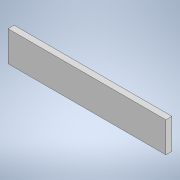
# Autodesk Inventor part: GroundShorttrack
Saved by Autodesk Inventor 2021 (Build 250183000, 183)
## iProperties
Created: 2022-07-02
Part Number: GroundShorttrack
Material: 一般
Document SubType Name: Modeling
Designer: tazak
Density: 1 g/cm^3
Appearance: 既定
Author: tazak
Autodesk Inventor part; units mm, degrees
ref_plane "YZ Plane" through (0, 0, 0) normal (1, 0, 0) x (0, 1, 0)
ref_plane "XZ Plane" through (0, 0, 0) normal (0, 1, 0) x (-1, 0, 0)
ref_plane "XY Plane" through (0, 0, 0) normal (0, 0, 1) x (1, 0, 0)
sketch "スケッチ1" plane through (0, 0, 0) normal (0, 0, 1) x (1, 0, 0)
  line L0 (-1000, 2500) -> (25000, 2500)
  line L1 (25000, 2500) -> (25000, -2500)
  line L2 (25000, -2500) -> (-1000, -2500)
  line L3 (-1000, -2500) -> (-1000, 2500)
  point P0 (0, 0)
  point P1 (-1000, 0)
  dimension "d0" = 1000
  dimension "d1" = 25000
  dimension "d2" = 5000
  constraints: 8 end point, 2 parallel, 1 horizontal, 1 horizontal alignment, 1 midpoint, 1 perpendicular
  measures "d0" distance from line of point (0, 0) L3
  measures "d1" distance from line of L1 point (0, 0)
  measures "d2" distance of L2.end L0.start
extrude "押し出し1" add sketch "スケッチ1" against normal blind 1000
